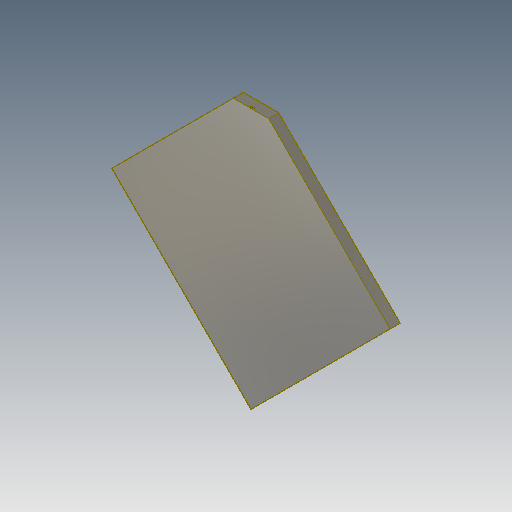
# Autodesk Inventor part: silvering
Saved by Autodesk Inventor 2020 (Build 240168000, 168)
## iProperties
Created: 2016-02-15
Part Number: silvering
Material: Silver
Document SubType Name: Modeling
Designer: sawai
Density: 10.49 g/cm^3
Appearance: Silver
Author: sawai
Autodesk Inventor part; units mm, degrees
note: some values were not read from the file. Left out: dimensions or parameters whose unit could not be read.
ref_plane "YZ Plane" through (0, 0, 0) normal (1, 0, 0) x (0, 1, 0)
ref_plane "XZ Plane" through (0, 0, 0) normal (0, 1, 0) x (-1, 0, 0)
ref_plane "XY Plane" through (0, 0, 0) normal (0, 0, 1) x (1, 0, 0)
sketch "Sketch1" plane through (0, 0, 0) normal (0, 0, 1) x (1, 0, 0)
  line L0 (-141.4214, 0) -> (-17.9605, 123.4608)
  line L1 (17.9605, 123.4608) -> (141.4214, 0)
  line L2 (141.4214, 0) -> (0, -141.4214)
  line L3 (0, -141.4214) -> (-141.4214, 0)
  line L4 (-141.4214, 0) -> (141.4214, 0) construction
  line L5 (0, 141.4214) -> (0, -141.4214) construction
  line L6 (17.9605, 123.4608) -> (-17.9605, 123.4608)
  line L7 (-18.0434, 123.6608) -> (18.0434, 123.6608)
  line L8 (18.0434, 123.6608) -> (141.7042, 0)
  line L9 (141.7042, 0) -> (0, -141.7042)
  line L10 (0, -141.7042) -> (-141.7042, 0)
  line L11 (-141.7042, 0) -> (-18.0434, 123.6608)
  point P0 (0, 0)
  dimension "d0" = 200
  dimension "d1" = 200
  dimension "d7" = 25.4
  dimension "d8" = 25.4
  dimension "d9" = 0.2
  constraints: 24 end point, 4 parallel, 2 midpoint, 2 perpendicular, 2 point on line, 1 horizontal, 4 other
  measures "d0" distance of L5.start L1.end
  measures "d1" distance between parallel lines of L3 L1
  measures "d7" distance of L1.start L5.start
  measures "d8" distance of L0.end L5.start
  measures "d9" distance between parallel lines of L0 L11
extrude "Extrusion1" add sketch "Sketch1" along normal mid plane 10
sketch "Sketch4" plane through (-18.0434, 123.6608, 5) normal (0, 1, 0) x (1, 0, 0)
  line L0 (16.0434, 0) -> (20.0434, 0)
  line L1 (20.0434, 0) -> (20.0434, 2)
  line L2 (20.0434, 2) -> (16.0434, 2)
  line L3 (16.0434, 2) -> (16.0434, 0)
  line L4 (36.0867, 0) -> (0, 0) projected
  point P0 (18.0434, 5)
  point P1 (18.0434, 0)
  dimension "d16" = 4
  dimension "d17" = 2
  constraints: 8 end point, 2 midpoint, 2 parallel, 1 horizontal, 1 perpendicular
  measures "d16" distance of L1.end L2.end
  measures "d17" distance of L2.end L0.start
extrude "Extrusion3" cut sketch "Sketch4" against normal up to surface (0.2 mm away)
sketch "Sketch2" plane through (0, 0, 5) normal (0, 0, 1) x (1, 0, 0)
  line L0 (141.7042, 0) -> (0, -141.7042) projected
  line L1 (18.0434, 123.6608) -> (141.7042, 0) projected
  line L2 (-18.0434, 123.6608) -> (18.0434, 123.6608) projected
  line L3 (-141.7042, 0) -> (-18.0434, 123.6608) projected
  line L4 (0, -141.7042) -> (-141.7042, 0) projected
extrude "Extrusion2" add sketch "Sketch2" along normal blind 0.2
mirror "Mirror1" about plane through (0, 0, 0) normal (0, 0, 1) of "Extrusion2"
equation "\"d0\" = ScintillatorWidth"
equation "\"d1\" = ScintillatorHeight"
equation "\"d7\" = cornerChamfer"
equation "\"d8\" = d7"
equation "\"d9\" = silveringThickness"
equation "\"d3\" = ScintillatorThickness"
equation "\"d5\" = silveringThickness"
equation "\"ScintillatorThickness\" = 10"
equation "\"OpticalFiberClearence\" = 0.15"
equation "\"ScintillatorEdgeClearence\" = 3"
equation "\"ScintillatorWidth\" = 200"
equation "\"ScintillatorHeight\" = 200"
equation "\"ShallowTrackDepth\" = 1.3"
equation "\"DeepTrackDepth\" = 5.571"
equation "\"FiberEdgeOffsett\" = 5"
equation "\"LoopLargeTrackRatio\" = 1.5"
equation "\"FiberSensorClerence\" = 0.5"
equation "\"MountingScrewOffsett\" = 9"
equation "\"FoilThickness\" = 0.2"
equation "\"silveringThickness\" = 0.2"
equation "\"mppcMountDepth\" = 6.35"
equation "\"opticalFiberClearence\" = 0.071"
equation "\"scintillatorEdgeClearence\" = 3"
equation "\"fiberEdgeOffsett\" = 5"
equation "\"shallowTrackDepth\" = 1.142"
equation "\"deepTrackDepth\" = 5.571"
equation "\"opticalFiberDiameter\" = 1"
equation "\"mountingSpacing\" = 18"
equation "\"cornerChamfer\" = 25.4"
equation "\"SmallTrackDiameter\" = 175"
body "Solid1"
